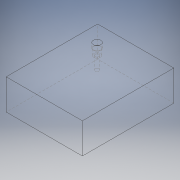
# Autodesk Inventor part: Thermocyler_Block_Test
Saved by Autodesk Inventor 2018 (Build 220112000, 112)
## iProperties
Part Number: Thermocyler_Block_Test
Material: Generic
Document SubType Name: Modeling
Designer: Intel
Appearance: Generic
Author: Intel
Autodesk Inventor part; units mm, degrees
ref_plane "YZ Plane" through (0, 0, 0) normal (1, 0, 0) x (0, 1, 0)
ref_plane "XZ Plane" through (0, 0, 0) normal (0, 1, 0) x (-1, 0, 0)
ref_plane "XY Plane" through (0, 0, 0) normal (0, 0, 1) x (1, 0, 0)
sketch "Sketch1" plane through (0, 0, 0) normal (0, 0, 1) x (1, 0, 0)
  line L0 (0, 0) -> (63.5, 0)
  line L1 (63.5, 0) -> (63.5, -25.4)
  line L2 (63.5, -25.4) -> (0, -25.4)
  line L3 (0, -25.4) -> (0, 0)
  dimension "d0" = 63.5
  dimension "d1" = 25.4
  constraints: 8 end point, 2 parallel, 1 horizontal, 1 perpendicular
  measures "d0" distance of L1.end L2.end
  measures "d1" distance of L0.end L1.end
extrude "Extrusion1" add sketch "Sketch1" along normal blind 76.2
sketch "Sketch2" plane through (0, 0, 0) normal (0, 1, 0) x (1, 0, 0)
  circle A0 centre (13.1221, -13.5403) radius 1.6574
  circle A1 centre (13.1221, -13.5403) radius 3.1433
  circle A2 centre (13.1221, -13.5403) radius 2.794
  point P0 (0, 0)
  point P1 (22.0121, -13.5403)
  point P2 (35.874, -13.5403)
  point P3 (13.1221, -22.4303)
  point P4 (22.0121, -22.4303)
  point P5 (13.1221, -22.4303)
  dimension "d4" = 3.3147
  dimension "d5" = 6.2865
  dimension "d6" = 5.588
  dimension "d22" = 8.89
  dimension "d23" = 8.89
  dimension "d24" = 8.89
  constraints: 4 coincident, 3 centre point
  measures "d4" diameter of A0
  measures "d5" diameter of A1
  measures "d6" diameter of A2
  measures "d22" distance of A0.centre point (13.122, -22.43)
  measures "d23" distance of point (22.012, -22.43) point (22.012, -13.54)
  measures "d24" distance of A0.centre point (22.012, -13.54)
extrude "Extrusion2" cut sketch "Sketch2" against normal blind 19.812 contours A0
extrude "Extrusion3" cut sketch "Sketch2" against normal blind 9.398 contours A2
extrude "Extrusion4" cut sketch "Sketch2" against normal blind 4.1148 contours A1
fillet "Fillet1" [suppressed]
loft "Loft1" [suppressed]
body "Solid1"
